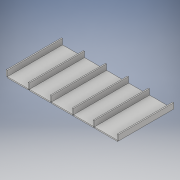
# Autodesk Inventor part: toboggan
Saved by Autodesk Inventor 2019 (Build 230136000, 136)
## iProperties
Created: 2018-11-20
Part Number: toboggan
Material: Générique
Document SubType Name: Modeling
Designer: pouey
Density: 1 g/cm^3
Appearance: Par défaut
Author: pouey
Autodesk Inventor part; units mm, degrees
ref_plane "YZ Plane" through (0, 0, 0) normal (1, 0, 0) x (0, 1, 0)
ref_plane "XZ Plane" through (0, 0, 0) normal (0, 1, 0) x (-1, 0, 0)
ref_plane "XY Plane" through (0, 0, 0) normal (0, 0, 1) x (1, 0, 0)
sketch "Esquisse1" plane through (0, 0, 0) normal (0, 1, 0) x (-1, 0, 0)
  line L0 (0, 0) -> (200, 0)
  line L1 (200, 0) -> (200, -100)
  line L2 (200, -100) -> (0, -100)
  line L3 (0, -100) -> (0, 0)
  line L4 (162, 0) -> (160, 0)
  line L5 (160, 0) -> (160, -100)
  line L6 (160, -100) -> (162, -100)
  line L7 (162, -100) -> (162, 0)
  line L8 (122, 0) -> (120, 0)
  line L9 (120, 0) -> (120, -100)
  line L10 (120, -100) -> (122, -100)
  line L11 (122, -100) -> (122, 0)
  line L12 (82, 0) -> (80, 0)
  line L13 (80, 0) -> (80, -100)
  line L14 (80, -100) -> (82, -100)
  line L15 (82, -100) -> (82, 0)
  line L16 (42, 0) -> (44, 0)
  line L17 (44, 0) -> (44, -100)
  line L18 (44, -100) -> (42, -100)
  line L19 (42, -100) -> (42, 0)
  line L20 (200, 0) -> (0, 0)
  line L21 (0, 0) -> (0, -100)
  line L22 (0, -100) -> (200, -100)
  line L23 (200, -100) -> (200, 0)
  line L24 (200, 0) -> (202, 0)
  line L25 (202, 0) -> (202, -100)
  line L26 (202, -100) -> (200, -100)
  line L27 (200, -100) -> (200, 0)
  dimension "d0" = 100
  dimension "d1" = 200
  dimension "d2" = 38
  dimension "d3" = 2
  dimension "d4" = 38
  dimension "d5" = 2
  dimension "d6" = 38
  dimension "d7" = 2
  dimension "d8" = 38
  dimension "d9" = 2
  dimension "d14" = 2
  dimension "d15" = 100
  constraints: 56 end point, 14 parallel, 8 point on line, 7 horizontal, 7 perpendicular
  measures "d0" distance of L0.end L1.end
  measures "d1" distance between parallel lines of L3 L1
  measures "d2" distance between parallel lines of L1 L7
  measures "d3" distance between parallel lines of L7 L5
  measures "d4" distance between parallel lines of L11 L5
  measures "d5" distance between parallel lines of L9 L11
  measures "d6" distance between parallel lines of L15 L9
  measures "d7" distance between parallel lines of L15 L13
  measures "d8" distance between parallel lines of L19 L13
  measures "d9" distance between parallel lines of L17 L19
  measures "d14" distance between parallel lines of L1 L25
  measures "d15" distance between parallel lines of L24 L26
extrude "Extrusion1" add sketch "Esquisse1" along normal blind 10 contours L0 L17 L2 L19 | L0 L15 L2 L13 | L0 L11 L2 L9 | L0 L7 L2 L5
extrude "Extrusion2" add sketch "Esquisse1" against normal blind 2 contours L0 L19 L2 L3 | L0 L13 L2 L17 | L0 L9 L2 L15 | L0 L5 L2 L11 | L0 L1 L2 L7
extrude "Extrusion3" add sketch "Esquisse1" along normal blind 10 contours L24 L25 L26 L1
sketch "Esquisse2" plane through (0, 0, 0) normal (0, 1, 0) x (1, 0, 0)
  line L0 (0, 100) -> (2, 100)
  line L1 (2, 100) -> (2, 0)
  line L2 (2, 0) -> (0, 0)
  line L3 (0, 0) -> (0, 100)
  dimension "d18" = 100
  dimension "d19" = 2
  constraints: 8 end point, 2 parallel, 1 horizontal, 1 perpendicular
  measures "d18" distance between parallel lines of L2 L0
  measures "d19" distance between parallel lines of L3 L1
extrude "Extrusion4" add sketch "Esquisse2" along normal blind 10
